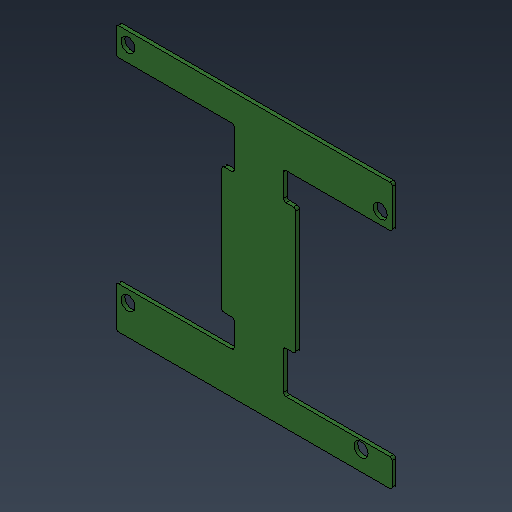
# Autodesk Inventor part: PCB_InterfaceBoard
Saved by Autodesk Inventor 2026.2 (Build 302298010, 298A)
## iProperties
Created: 2026-04-14
Part Number: PCB_InterfaceBoard
Material: Generic
Document SubType Name: Modeling
Designer: szymo
Density: 1 g/cm^3
Appearance: Default(1)
Author: szymo
Autodesk Inventor part; units mm, degrees
ref_plane "YZ Plane" through (0, 0, 0) normal (1, 0, 0) x (0, 1, 0)
ref_plane "XZ Plane" through (0, 0, 0) normal (0, 1, 0) x (-1, 0, 0)
ref_plane "XY Plane" through (0, 0, 0) normal (0, 0, 1) x (1, 0, 0)
sketch "Sketch1" plane through (0, 0, 0) normal (0, 0, 1) x (1, 0, 0)
  line L0 (12.6749, 0) -> (12.6749, 3) projected
  line L1 (12.6749, 3) -> (20.628, 3) projected
  line L2 (20.628, 3) -> (20.628, 0) projected
  line L3 (20.628, 0) -> (59.3371, 0) projected
  line L4 (59.3371, 0) -> (59.3371, 9.3) projected
  line L5 (59.3371, 9.3) -> (0, 9.3) projected
  line L6 (0, 3) -> (0, 9.3) projected
  line L7 (0, 3) -> (4.1896, 3) projected
  line L8 (4.1896, 3) -> (4.1896, 0) projected
  line L9 (4.1896, 0) -> (12.6749, 0) projected
  line L10 (41.8802, -41.4) -> (41.8802, -38.4) projected
  line L11 (0, -38.4) -> (41.8802, -38.4) projected
  line L12 (0, -38.4) -> (0, -47.7) projected
  line L13 (0, -47.7) -> (59.3371, -47.7) projected
  line L14 (59.3371, -41.4) -> (59.3371, -47.7) projected
  line L15 (59.3371, -41.4) -> (57.1475, -41.4) projected
  line L16 (57.1475, -41.4) -> (57.1475, -38.4) projected
  line L17 (48.6622, -38.4) -> (57.1475, -38.4) projected
  line L18 (48.6622, -38.4) -> (48.6622, -41.4) projected
  line L19 (48.6622, -41.4) -> (41.8802, -41.4) projected
  line L20 (39.0735, -33.15) -> (39.0735, -5.25)
  line L21 (39.0735, -5.25) -> (39.9371, -5.25)
  line L22 (39.9371, -5.25) -> (39.9371, -33.15)
  line L23 (39.9371, -33.15) -> (39.0735, -33.15)
  line L24 (22.2636, -5.25) -> (22.2636, -33.15)
  line L25 (22.2636, -33.15) -> (21.4, -33.15)
  line L26 (21.4, -33.15) -> (21.4, -5.25)
  line L27 (21.4, -5.25) -> (22.2636, -5.25)
  line L28 (21.4, 0) -> (21.4, -38.4)
  line L29 (16.4787, 3) -> (18.0543, 3)
  line L30 (39.9371, -38.4) -> (39.9371, 0)
  line L31 (39.9371, 0) -> (62.3371, 0)
  line L32 (59.1371, 9.1) -> (59.1371, 0.2)
  line L33 (59.1371, 0.2) -> (35.9371, 0.2)
  line L34 (35.9371, 0.2) -> (35.9371, -5.75)
  line L35 (35.9371, -5.75) -> (38.5735, -5.75)
  line L36 (38.5735, -5.75) -> (38.5735, -32.65)
  line L37 (35.9371, -32.65) -> (35.9371, -41.6)
  line L38 (35.9371, -41.6) -> (59.1371, -41.6)
  line L39 (59.1371, -41.6) -> (59.1371, -47.5)
  line L40 (59.1371, -47.5) -> (0.2, -47.5)
  line L41 (0.2, -47.5) -> (0.2, -38.6)
  line L42 (0.2, -38.6) -> (25.4, -38.6)
  line L43 (25.4, -38.6) -> (25.4, -32.65)
  line L44 (25.4, -32.65) -> (22.7636, -32.65)
  line L45 (22.7636, -32.65) -> (22.7636, -5.75)
  line L46 (22.7636, -5.75) -> (25.4, -5.75)
  line L47 (25.4, -5.75) -> (25.4, 3.2)
  line L48 (25.4, 3.2) -> (0.2, 3.2)
  line L49 (0.2, 3.2) -> (0.2, 9.1)
  line L50 (0.2, 9.1) -> (59.1371, 9.1)
  line L51 (38.5735, -32.65) -> (35.9371, -32.65)
  circle A0 centre (2.75, -41.15) radius 1.75 projected
  circle A1 centre (52.4871, -43.4) radius 1.75 projected
  circle A2 centre (56.5871, 2.75) radius 1.75 projected
  circle A3 centre (2.75, 6.55) radius 1.75 projected
  circle A4 centre (56.5871, 2.75) radius 1.5
  circle A5 centre (52.4871, -43.4) radius 1.5
  circle A6 centre (2.75, -41.15) radius 1.5
  circle A7 centre (2.75, 6.55) radius 1.5
  point P0 (0, 0)
  point P1 (35.9371, 0)
  point P2 (35.9371, -38.4)
  dimension "d1" = 0.2
  dimension "d3" = 0.2
  dimension "d4" = 0.2
  dimension "d5" = 0.2
  dimension "d6" = 0.2
  dimension "d7" = 0.2
  dimension "d8" = 0.2
  dimension "d9" = 0.2
  dimension "d10" = 0.2
  dimension "d11" = 0.2
  dimension "d16" = 0.5
  dimension "d17" = 0.5
  dimension "d18" = 4
  dimension "d19" = 0.5
  dimension "d20" = 0.5
  dimension "d21" = 0.5
  dimension "d22" = 0.5
  dimension "d23" = 4
  dimension "d24" = 4
  dimension "d25" = 4
  dimension "d29" = 3
  dimension "d30" = 3
  dimension "d31" = 3
  dimension "d32" = 3
  constraints: 65 end point, 11 perpendicular, 9 vertical, 8 horizontal, 4 centre point, 4 coincident, 3 parallel, 13 other
  measures "d1" distance between parallel lines of L33 L31
  measures "d3" distance between parallel lines of L4 L32
  measures "d4" distance between parallel lines of L5 L50
  measures "d5" distance between parallel lines of L6 L49
  measures "d6" distance between parallel lines of L7 L48
  measures "d7" distance between parallel lines of L11 L42
  measures "d8" distance between parallel lines of L12 L41
  measures "d9" distance between parallel lines of L15 L38
  measures "d10" distance between parallel lines of L14 L39
  measures "d11" distance between parallel lines of L13 L40
  measures "d16" distance between parallel lines of L45 L24
  measures "d17" distance between parallel lines of L20 L36
  measures "d18" distance between parallel lines of L47 L28
  measures "d19" distance between parallel lines of L46 L27
  measures "d20" distance between parallel lines of L35 L21
  measures "d21" distance between parallel lines of L44 L25
  measures "d22" distance between parallel lines of L23 L51
  measures "d23" distance between parallel lines of L34 L30
  measures "d24" distance between parallel lines of L37 L30
  measures "d25" distance between parallel lines of L28 L43
  measures "d29" diameter of A4
  measures "d30" diameter of A5
  measures "d31" diameter of A6
  measures "d32" diameter of A7
extrude "Extrusion1" add sketch "Sketch1" along normal blind 0.8 contours L47 L48 L49 L50 L32 L33 L34 L3 | L3 L34 L35 L36 L51 L37 L11 L43 L44 L45 L46 L47 | L11 L37 L38 L39 L40 L41 L42 L43 | A0 | A1 | A2 | A3
fillet "Fillet1" radius 0.5 20 edges at (59.1371, -47.5, 0.4) (59.1371, -41.6, 0.4) (0.2, -47.5, 0.4) (0.2, -38.6, 0.4) (25.4, -38.6, 0.4) (25.4, -32.65, 0.4) (22.7636, -32.65, 0.4) (22.7636, -5.75, 0.4) (25.4, -5.75, 0.4) (25.4, 3.2, 0.4) (0.2, 3.2, 0.4) (0.2, 9.1, 0.4) (59.1371, 9.1, 0.4) (59.1371, 0.2, 0.4) (35.9371, 0.2, 0.4) (35.9371, -5.75, 0.4) (38.5735, -5.75, 0.4) (38.5735, -32.65, 0.4) (35.9371, -32.65, 0.4) (35.9371, -41.6, 0.4)
equation "\"d3\" = d1"
equation "\"d4\" = d1"
equation "\"d5\" = d1"
equation "\"d6\" = d1"
equation "\"d7\" = d1"
equation "\"d8\" = d1"
equation "\"d9\" = d1"
equation "\"d10\" = d1"
equation "\"d11\" = d1"
equation "\"d16\" = d17"
equation "\"d18\" = d23"
equation "\"d19\" = d20"
equation "\"d21\" = d20"
equation "\"d22\" = d20"
equation "\"d24\" = d23"
equation "\"d25\" = d23"
equation "\"d30\" = d29"
equation "\"d31\" = d29"
equation "\"d32\" = d29"
body "Solid1"
